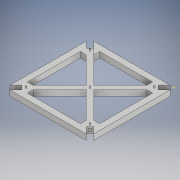
# Autodesk Inventor part: Frame
Saved by Autodesk Inventor 2018 (Build 220112000, 112)
## iProperties
Created: 2017-04-26
Part Number: Frame
Material: Generic
Document SubType Name: Modeling
Designer: beesmerr13
Density: 1 g/cm^3
Appearance: Default
Author: beesmerr13
Autodesk Inventor part; units mm, degrees
ref_plane "YZ Plane" through (0, 0, 0) normal (1, 0, 0) x (0, 1, 0)
ref_plane "XZ Plane" through (0, 0, 0) normal (0, 1, 0) x (-1, 0, 0)
ref_plane "XY Plane" through (0, 0, 0) normal (0, 0, 1) x (1, 0, 0)
sketch "Sketch1" plane through (0, 0, 0) normal (0, 1, 0) x (-1, 0, 0)
  line L0 (0, -7.0711) -> (0, -142.9289)
  line L1 (7.0711, 0) -> (142.9289, 0)
  line L2 (150, -7.0711) -> (150, -142.9289)
  line L3 (142.9289, -150) -> (7.0711, -150)
  line L4 (139.3934, -10.6066) -> (135.8579, -14.1421)
  line L5 (135.8579, -14.1421) -> (132.3223, -10.6066)
  line L6 (132.3223, -10.6066) -> (135.8579, -14.1421)
  line L7 (135.8579, -14.1421) -> (139.3934, -17.6777)
  line L8 (139.3934, -17.6777) -> (150, -7.0711)
  line L9 (132.3223, -10.6066) -> (142.9289, 0)
  line L10 (139.3934, -139.3934) -> (135.8579, -135.8579)
  line L11 (135.8579, -135.8579) -> (132.3223, -139.3934)
  line L12 (132.3223, -139.3934) -> (142.9289, -150)
  line L13 (135.8579, -135.8579) -> (139.3934, -132.3223)
  line L14 (139.3934, -132.3223) -> (150, -142.9289)
  line L15 (10.6066, -139.3934) -> (14.1421, -135.8579)
  line L16 (14.1421, -135.8579) -> (10.6066, -132.3223)
  line L17 (10.6066, -132.3223) -> (14.1421, -135.8579)
  line L18 (14.1421, -135.8579) -> (17.6777, -139.3934)
  line L19 (17.6777, -139.3934) -> (7.0711, -150)
  line L20 (10.6066, -132.3223) -> (0, -142.9289)
  line L21 (10.6066, -10.6066) -> (14.1421, -14.1421)
  line L22 (14.1421, -14.1421) -> (10.6066, -17.6777)
  line L23 (10.6066, -17.6777) -> (14.1421, -14.1421)
  line L24 (14.1421, -14.1421) -> (17.6777, -10.6066)
  line L25 (7.0711, 0) -> (17.6777, -10.6066)
  line L26 (10.6066, -17.6777) -> (0, -7.0711)
  line L27 (132.3223, -10.6066) -> (75, -67.9289)
  line L28 (67.9289, -75) -> (10.6066, -132.3223)
  line L29 (132.3223, -10.6066) -> (17.6777, -10.6066)
  line L30 (139.3934, -17.6777) -> (139.3934, -132.3223)
  line L31 (132.3223, -139.3934) -> (17.6777, -139.3934)
  line L32 (10.6066, -132.3223) -> (10.6066, -17.6777)
  line L33 (139.3934, -10.6066) -> (135.8579, -14.1421)
  line L34 (14.1421, -135.8579) -> (0, -150)
  line L35 (10.6066, -10.6066) -> (14.1421, -14.1421)
  line L36 (135.8579, -135.8579) -> (139.3934, -139.3934)
  line L37 (139.3934, -132.3223) -> (82.0711, -75)
  line L38 (75, -67.9289) -> (17.6777, -10.6066)
  line L39 (10.6066, -17.6777) -> (67.9289, -75)
  line L40 (75, -82.0711) -> (132.3223, -139.3934)
  line L41 (139.3934, -17.6777) -> (82.0711, -75)
  line L42 (75, -82.0711) -> (17.6777, -139.3934)
  point P0 (0, 0)
  dimension "d0" = 150
  constraints: 86 end point, 27 perpendicular, 13 point on line, 8 parallel, 3 collinear, 1 horizontal, 1 vertical
  measures "d0" distance of point (0, 0) L34.end
extrude "Extrusion1" add sketch "Sketch1" along normal blind 10 contours L26 L32 L20 L0 | L22 L24 L38 L27 L5 L7 L41 L37 L13 L11 L40 L42 L18 L16 L28 L39 | L25 L1 L9 L29 | L31 L12 L3 L19 | L8 L2 L14 L30
sketch "Sketch2" plane through (0, 10, 0) normal (0, 1, 0) x (1, 0, 0)
  line L0 (-17.6777, 10.6066) -> (-27.6777, 10.6066)
  line L1 (-17.6777, 10.6066) -> (-132.3223, 10.6066) projected
  line L2 (-27.6777, 10.6066) -> (-27.6777, 20.6066)
  line L3 (-75, 67.9289) -> (-17.6777, 10.6066) projected
  line L4 (-10.6066, 17.6777) -> (-67.9289, 75) projected
  line L5 (-20.6066, 27.6777) -> (-10.6066, 27.6777)
  line L6 (-10.6066, 27.6777) -> (-10.6066, 17.6777)
  line L7 (-10.6066, 132.3223) -> (-10.6066, 17.6777) projected
  line L8 (-132.3223, 10.6066) -> (-75, 67.9289) projected
  line L9 (-132.3223, 10.6066) -> (-122.3223, 10.6066)
  line L10 (-122.3223, 10.6066) -> (-122.3223, 20.6066)
  line L11 (-122.3223, 20.6066) -> (-129.3934, 27.6777)
  line L12 (-82.0711, 75) -> (-139.3934, 17.6777) projected
  line L13 (-139.3934, 27.6777) -> (-129.3934, 27.6777)
  line L14 (-139.3934, 17.6777) -> (-139.3934, 132.3223) projected
  line L15 (-139.3934, 27.6777) -> (-139.3934, 17.6777)
  line L16 (-139.3934, 17.6777) -> (-129.3934, 27.6777)
  line L17 (-132.3223, 10.6066) -> (-122.3223, 20.6066)
  line L18 (-139.3934, 132.3223) -> (-139.3934, 122.3223)
  line L19 (-139.3934, 122.3223) -> (-129.3934, 122.3223)
  line L20 (-139.3934, 132.3223) -> (-82.0711, 75) projected
  line L21 (-129.3934, 122.3223) -> (-122.3223, 129.3934)
  line L22 (-75, 82.0711) -> (-132.3223, 139.3934) projected
  line L23 (-122.3223, 129.3934) -> (-122.3223, 139.3934)
  line L24 (-132.3223, 139.3934) -> (-17.6777, 139.3934) projected
  line L25 (-122.3223, 139.3934) -> (-132.3223, 139.3934)
  line L26 (-17.6777, 139.3934) -> (-75, 82.0711) projected
  line L27 (-17.6777, 139.3934) -> (-27.6777, 139.3934)
  line L28 (-27.6777, 129.3934) -> (-27.6777, 139.3934)
  line L29 (-27.6777, 129.3934) -> (-20.6065, 122.3222)
  line L30 (-20.6065, 122.3222) -> (-10.6066, 122.3222)
  line L31 (-10.6066, 132.3223) -> (-20.6065, 122.3222)
  line L32 (-10.6066, 17.6777) -> (-20.6066, 27.6777)
  line L33 (-27.6777, 20.6066) -> (-17.6777, 10.6066)
  line L34 (-10.6066, 17.6777) -> (-10.6066, 27.6777)
  line L35 (-20.6066, 27.6777) -> (-10.6066, 17.6777)
  point P0 (0, 0)
  dimension "d9" = 10
  dimension "d10" = 10
  dimension "d11" = 10
  constraints: 50 end point, 17 point on line, 9 perpendicular, 5 collinear, 1 horizontal, 1 parallel
  measures "d9" distance of L0.start L0.end
  measures "d10" distance of L1.end L9.end
  measures "d11" distance of L14.end L18.end
extrude "Extrusion2" add sketch "Sketch2" against normal blind 10 contours L6 L4 L5 | L31 L7 L30 | L22 L24 L23 | L12 L14 L13 | L0 L2 L3 | L1 L8 L10 | L19 L14 L20 | L28 L24 L26
sketch "Sketch3" plane through (0, 10, 0) normal (0, 1, 0) x (1, 0, 0)
  line L0 (-67.9289, 75) -> (-10.6066, 132.3223) projected
  line L1 (-82.0711, 75) -> (-75, 67.9289)
  circle A0 centre (-75, 75) radius 1.25
  line L2 (-75, 82.0711) -> (-122.3223, 129.3934) projected
  line L3 (-82.0711, 75) -> (-129.3934, 27.6777) projected
  line L4 (-17.6777, 10.6066) -> (-10.6066, 17.6777) projected
  line L5 (-14.1421, 14.1421) -> (-17.6777, 10.6066)
  line L6 (-17.6777, 10.6066) -> (-14.1421, 14.1421)
  line L7 (-14.1421, 14.1421) -> (-17.6777, 10.6066)
  line L8 (-20.6066, 27.6777) -> (-67.9289, 75) projected
  line L9 (-10.6066, 132.3223) -> (-17.6777, 139.3934) projected
  circle A1 centre (-132.226, 17.774) radius 1.25
  circle A2 centre (-132.136, 132.136) radius 1.25
  circle A3 centre (-17.6777, 132.3223) radius 1.25
  circle A4 centre (-17.6777, 17.6777) radius 1.25
  point P0 (0, 0)
  dimension "d14" = 2.5
  dimension "d21" = 2.5
  constraints: 8 end point, 5 centre point, 3 collinear, 1 midpoint, 1 perpendicular
  measures "d14" diameter of A0
  measures "d21" diameter of A3
extrude "Extrusion3" add sketch "Sketch3" along normal blind 2.5
sketch "Sketch4" plane through (-10.6066, 0, -17.6777) normal (0.7071, 0, 0.7071) x (0.7071, 0, -0.7071)
  line L0 (-5, 0) -> (-5, 2.5)
  line L1 (-5, 2.5) -> (-2.5, 2.5)
  line L2 (-2.5, 2.5) -> (-2.5, 7.5)
  line L3 (-2.5, 7.5) -> (-7.5, 7.5)
  line L4 (-7.5, 7.5) -> (-7.5, 2.5)
  line L5 (-7.5, 2.5) -> (-5, 2.5)
  dimension "d25" = 2.5
  dimension "d26" = 2.5
  dimension "d27" = 5
  dimension "d28" = 5
  constraints: 12 end point, 5 perpendicular, 1 point on line, 1 vertical
  measures "d25" distance of L0.start L0.end
  measures "d26" distance of L0.end L1.end
  measures "d27" distance of L1.end L2.end
  measures "d28" distance of L2.end L3.end
extrude "Extrusion4" cut sketch "Sketch4" against normal blind 15
sketch "Sketch5" plane through (-132.3223, 0, -10.6066) normal (-0.7071, 0, 0.7071) x (0.7071, 0, 0.7071)
  line L0 (0, 0) -> (0, 10) projected
  line L1 (0, 0) -> (0, 5)
  line L2 (0, 5) -> (-2.5, 5)
  line L3 (-2.5, 5) -> (0, 5)
  line L4 (-2.5, 5) -> (-2.5, 7.5)
  line L5 (-2.5, 7.5) -> (-7.5, 7.5)
  line L6 (-7.5, 7.5) -> (-7.5, 2.5)
  line L7 (-7.5, 2.5) -> (-2.5, 2.5)
  line L8 (-2.5, 2.5) -> (-2.5, 5)
  point P0 (101.066, 0)
  dimension "d31" = 5
  dimension "d32" = 2.5
  dimension "d33" = 2.5
  dimension "d34" = 5
  constraints: 16 end point, 6 perpendicular, 1 collinear, 1 midpoint, 1 point on line
  measures "d31" distance of L0.start L1.end
  measures "d32" distance of L1.end L2.end
  measures "d33" distance of L2.end L4.end
  measures "d34" distance of L4.end L5.end
extrude "Extrusion5" cut sketch "Sketch5" against normal blind 15
sketch "Sketch6" plane through (-139.3934, 0, -132.3223) normal (-0.7071, 0, -0.7071) x (-0.7071, 0, 0.7071)
  line L0 (-5, 0) -> (-5, 2.5)
  line L1 (-7.5, 2.5) -> (-2.5, 2.5) projected
  line L2 (-5, 2.5) -> (-2.5, 2.5)
  line L3 (-2.5, 2.5) -> (-2.5, 7.5) projected
  line L4 (-2.5, 2.5) -> (-2.5, 7.5)
  line L5 (-2.5, 7.5) -> (-7.5, 7.5) projected
  line L6 (-2.5, 7.5) -> (-7.5, 7.5)
  line L7 (-7.5, 7.5) -> (-7.5, 2.5)
  line L8 (-7.5, 2.5) -> (-5, 2.5)
  dimension "d37" = 2.5
  constraints: 12 end point, 2 collinear, 1 perpendicular, 1 vertical
  measures "d37" distance of L0.start L0.end
extrude "Extrusion6" cut sketch "Sketch6" against normal blind 15
sketch "Sketch7" plane through (-17.6777, 0, -139.3934) normal (0.7071, 0, -0.7071) x (-0.7071, 0, -0.7071)
  line L0 (0, 0) -> (-5, 0)
  line L1 (-10, 0) -> (0, 0) projected
  line L2 (-5, 0) -> (-5, 2.5)
  line L3 (-7.5, 2.5) -> (-2.5, 2.5) projected
  line L4 (-2.5, 2.5) -> (-2.5, 7.5) projected
  line L5 (-2.5, 2.5) -> (-2.5, 7.5)
  line L6 (-2.5, 7.5) -> (-7.5, 7.5) projected
  line L7 (-2.5, 7.5) -> (-7.5, 7.5)
  line L8 (-7.5, 7.5) -> (-7.5, 2.5) projected
  line L9 (-7.5, 7.5) -> (-7.5, 2.5)
  line L10 (-7.5, 2.5) -> (-5, 2.5)
  point P0 (-111.066, 0)
  dimension "d40" = 5
  constraints: 12 end point, 4 collinear, 2 midpoint
  measures "d40" distance of L0.start L0.end
extrude "Extrusion7" cut sketch "Sketch7" against normal blind 15
sketch "Sketch8" plane through (0, 10, 0) normal (0, 1, 0) x (1, 0, 0)
  point P0 (0, 0)
body "Solid1"
